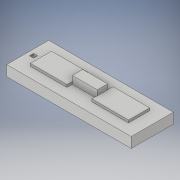
# Autodesk Inventor part: ODS_Enclosure_Bottom_V2D4
Saved by Autodesk Inventor 2017 (Build 210142000, 142)
## iProperties
Created: 2017-12-29
Part Number: ODS_Enclosure_Bottom_V2D4
Material: Generic
Document SubType Name: Modeling
Designer: Tripl_000
Density: 1 g/cm^3
Appearance: Default
Author: Tripl_000
Autodesk Inventor part; units mm, degrees
ref_plane "YZ Plane" through (0, 0, 0) normal (1, 0, 0) x (0, 1, 0)
ref_plane "XZ Plane" through (0, 0, 0) normal (0, 1, 0) x (-1, 0, 0)
ref_plane "XY Plane" through (0, 0, 0) normal (0, 0, 1) x (1, 0, 0)
sketch "Sketch1" plane through (0, 0, 0) normal (1, 0, 0) x (0, 1, 0)
  line L0 (1.4605, 13.081) -> (-1.4605, 13.081)
  line L1 (-1.4605, 13.081) -> (-1.4605, -13.081)
  line L2 (-1.4605, -13.081) -> (1.4605, -13.081)
  line L3 (1.4605, -13.081) -> (1.4605, 13.081)
  line L4 (1.4605, 13.081) -> (-1.4605, -13.081) construction
  line L5 (-1.4605, 13.081) -> (1.4605, -13.081) construction
  point P0 (0, 0)
  dimension "d0" = 2.921
  dimension "d1" = 26.162
  constraints: 12 end point, 2 midpoint, 2 parallel, 1 horizontal, 1 perpendicular
  measures "d0" distance between parallel lines of L1 L3
  measures "d1" distance of L2.end L0.start
extrude "Extrusion1" add sketch "Sketch1" along normal blind 120.142
sketch "Sketch2" plane through (0, -1.4605, -13.081) normal (0, -1, 0) x (1, 0, 0)
  line L0 (0, 26.162) -> (120.142, 26.162) projected
  line L1 (75.311, 26.162) -> (44.831, 26.162)
  line L2 (44.831, 26.162) -> (44.831, 19.5072)
  line L3 (44.831, 19.5072) -> (75.311, 19.5072)
  line L4 (75.311, 19.5072) -> (75.311, 26.162)
  line L5 (-38.891, 13.081) -> (135.1376, 13.081)
  line L6 (0, 26.162) -> (0, 0) projected
  line L7 (44.831, 0) -> (44.831, 6.6548)
  line L8 (44.831, 6.6548) -> (75.311, 6.6548)
  line L9 (75.311, 6.6548) -> (75.311, 0)
  line L10 (75.311, 0) -> (44.831, 0)
  line L11 (0, 0) -> (120.142, 0) projected
  point P0 (0, 13.081)
  dimension "d4" = 44.831
  dimension "d5" = 30.48
  dimension "d6" = 6.6548
  constraints: 18 end point, 4 symmetric about line, 2 horizontal, 2 parallel, 1 collinear, 1 perpendicular, 1 point on line
  measures "d4" distance between parallel lines of L6 L2
  measures "d5" distance between parallel lines of L2 L4
  measures "d6" distance between parallel lines of L3 L0
extrude "Extrusion2" cut sketch "Sketch2" against normal through all
sketch "Sketch3" plane through (0, 1.4605, 13.081) normal (0, 1, 0) x (1, 0, 0)
  line L0 (75.311, 6.6548) -> (44.831, 6.6548) projected
  line L1 (75.311, 19.5072) -> (75.311, 26.162) projected
  line L2 (44.831, 6.6548) -> (75.311, 6.6548)
  line L3 (75.311, 6.6548) -> (75.311, 19.5072)
  line L4 (75.311, 19.5072) -> (44.831, 19.5072)
  line L5 (44.831, 19.5072) -> (44.831, 6.6548)
  point P0 (0, 13.081)
  constraints: 8 end point, 2 parallel, 1 horizontal, 1 perpendicular
extrude "Extrusion3" add sketch "Sketch3" along normal blind 6.35
ref_plane "Work Plane1" through (136.271, 0, 0) normal (1, 0, 0) x (0, 0, -1)
sketch "Sketch4" plane through (136.271, 0, 0) normal (1, 0, 0) x (0, 0, -1)
  line L0 (-44.45, -14.1605) -> (44.45, -14.1605)
  line L1 (44.45, -14.1605) -> (44.45, -1.4605)
  line L2 (44.45, -1.4605) -> (-44.45, -1.4605)
  line L3 (-44.45, -1.4605) -> (-44.45, -14.1605)
  line L4 (-44.45, -14.1605) -> (44.45, -1.4605) construction
  line L5 (44.45, -14.1605) -> (-44.45, -1.4605) construction
  line L6 (13.081, 1.4605) -> (-13.081, 1.4605) projected
  line L7 (13.081, -1.4605) -> (13.081, 1.4605) projected
  point P0 (0, 0)
  point P1 (0, -7.8105)
  dimension "d12" = 2.921
  dimension "d13" = 12.7
  dimension "d14" = 88.9
  dimension "d15" = 31.369
  constraints: 12 end point, 2 midpoint, 2 parallel, 1 horizontal, 1 perpendicular
  measures "d12" distance between parallel lines of L6 L2
  measures "d13" distance of L0.end L1.end
  measures "d14" distance between parallel lines of L1 L3
  measures "d15" distance between parallel lines of L7 L1
extrude "Extrusion4" add sketch "Sketch4" against normal blind 152.4
sketch "Sketch5" plane through (-16.129, 0, 0) normal (-1, 0, 0) x (0, 0, 1)
  line L0 (-2.54, -5.2705) -> (2.54, -5.2705)
  line L1 (2.54, -5.2705) -> (2.54, -10.3505)
  line L2 (2.54, -10.3505) -> (-2.54, -10.3505)
  line L3 (-2.54, -10.3505) -> (-2.54, -5.2705)
  line L4 (-2.54, -5.2705) -> (2.54, -10.3505) construction
  line L5 (2.54, -5.2705) -> (-2.54, -10.3505) construction
  line L6 (-44.45, -14.1605) -> (44.45, -14.1605) projected
  line L7 (44.45, -14.1605) -> (44.45, -1.4605) projected
  line L8 (-44.45, -1.4605) -> (44.45, -1.4605) projected
  point P0 (0, 0)
  point P1 (0, -7.8105)
  dimension "d19" = 41.91
  dimension "d20" = 5.08
  dimension "d21" = 5.08
  dimension "d22" = 3.81
  constraints: 12 end point, 2 midpoint, 2 parallel, 1 horizontal, 1 perpendicular
  measures "d19" distance between parallel lines of L7 L1
  measures "d20" distance of L0.start L0.end
  measures "d21" distance of L2.end L0.start
  measures "d22" distance between parallel lines of L8 L0
extrude "Extrusion5" cut sketch "Sketch5" against normal blind 9.779
sketch "Sketch6" plane through (136.271, -1.4605, 44.45) normal (0, 1, 0) x (1, 0, 0)
  line L0 (-152.4, 41.91) -> (-142.621, 41.91) projected
  line L1 (-147.701, 46.99) -> (-142.621, 46.99)
  line L2 (-142.621, 46.99) -> (-142.621, 41.91)
  line L3 (-142.621, 41.91) -> (-147.701, 41.91)
  line L4 (-147.701, 41.91) -> (-147.701, 46.99)
  line L5 (-147.701, 46.99) -> (-142.621, 41.91) construction
  line L6 (-142.621, 46.99) -> (-147.701, 41.91) construction
  point P0 (-136.271, 44.45)
  point P1 (-145.161, 44.45)
  dimension "d25" = 5.08
  dimension "d26" = 5.08
  constraints: 12 end point, 2 midpoint, 2 parallel, 1 horizontal, 1 perpendicular
  measures "d25" distance of L1.start L1.end
  measures "d26" distance of L3.end L1.start
extrude "Extrusion6" cut sketch "Sketch6" against normal up to surface (3.81 mm away)
fillet "Fillet1" radius 3.175 2 edges at (-6.35, -10.3505, 0) (-11.43, -5.2705, 0)
ref_plane "Work Plane2" through (75.311, 1.4605, 0) normal (0, 0, 1) x (1, 0, 0)
sketch "Sketch7" plane through (120.142, 0, 0) normal (1, 0, 0) x (0, 0, -1)
  line L0 (-13.081, -1.4605) -> (-12.954, -1.4605)
  line L1 (-12.954, -1.4605) -> (-12.954, 10.809)
  line L2 (-12.954, 10.809) -> (-13.081, 10.809)
  line L3 (-13.081, 10.809) -> (-13.081, -1.4605)
  point P0 (0, 0)
  dimension "d31" = 0.127
  constraints: 8 end point, 2 parallel, 1 horizontal, 1 perpendicular
  measures "d31" distance between parallel lines of L1 L3
extrude "Extrusion7" cut sketch "Sketch7" against normal through all
sketch "Sketch8" plane through (75.311, 1.4605, 6.4262) normal (1, 0, 0) x (0, 0, -1)
  line L0 (0, 0) -> (0, 6.35) projected
  line L1 (-6.5278, -2.921) -> (19.5072, -2.921) projected
  line L2 (0, 6.35) -> (0.0762, 6.35)
  line L3 (0.0762, 6.35) -> (0.0762, -2.921)
  line L4 (0.0762, -2.921) -> (0, -2.921)
  line L5 (0, -2.921) -> (0, 6.35)
  point P0 (6.4262, -1.4605)
  dimension "d34" = 0.0762
  constraints: 8 end point, 2 parallel, 1 horizontal, 1 perpendicular, 1 point on line
  measures "d34" distance between parallel lines of L3 L0
extrude "Extrusion8" cut sketch "Sketch8" against normal up to surface (30.48 mm away)
mirror "Mirror1" about plane through (75.311, 1.4605, 0) normal (0, 0, 1) of "Extrusion7", "Extrusion8"
sketch "Sketch9" plane through (136.271, -1.4605, 44.45) normal (0, 1, 0) x (1, 0, 0)
  line L0 (-152.4, 88.9) -> (-152.4, 0) projected
  line L1 (0, 0) -> (0, 88.9) projected
  line L2 (-152.4, 88.9) -> (0, 88.9)
  line L3 (0, 88.9) -> (0, 70.231)
  line L4 (0, 70.231) -> (-152.4, 70.231)
  line L5 (-152.4, 70.231) -> (-152.4, 88.9)
  point P0 (-136.271, 44.45)
  dimension "d37" = 18.669
  constraints: 8 end point, 2 parallel, 1 horizontal, 1 perpendicular, 1 point on line
  measures "d37" distance between parallel lines of L4 L2
extrude "Extrusion9" cut sketch "Sketch9" against normal through all
mirror "Mirror2" about plane through (75.311, 1.4605, 0) normal (0, 0, 1) of "Extrusion9"
body "Solid1"
